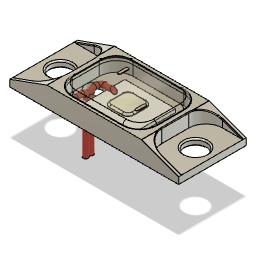
camera-imx335 (1) (Autodesk Fusion 360 archive; units mm, degrees)
design "LED light v3"
Autodesk Fusion 360 part; units mm, degrees
sketch "Sketch1" plane through (0, 0, 0) normal (0, 1, 0) x (1, 0, 0)
  line L0 (7.5, 6) -> (-7.5, 6)
  line L1 (-7.5, 6) -> (-7.5, -6)
  line L2 (-7.5, -6) -> (7.5, -6)
  line L3 (7.5, -6) -> (7.5, 6)
  line L4 (7.5, 6) -> (-7.5, -6) construction
  line L5 (-7.5, 6) -> (7.5, -6) construction
  dimension "d1" = 12
  dimension "d2" = 15
  constraint perpendicular L0 L1
  constraint parallel L0 L2
  constraint parallel L1 L3
  constraint horizontal L0
  constraint coincident L4 origin
  constraint coincident L5 origin
  measures "d1" distance of L0.end L1.end
  measures "d2" distance of L2.start L2.end L1
extrude "Extrude1" add sketch "Sketch1" along normal blind 1 makes body 1
sketch "Sketch2" plane through (0, 1, 0) normal (0, 1, 0) x (-1, 0, 0)
  line L0 (-7.5, 6) -> (-7.5, -6)
  line L1 (-7.5, -6) -> (7.5, -6)
  line L2 (7.5, -6) -> (7.5, 6)
  line L3 (7.5, 6) -> (-7.5, 6)
  line L4 (-3.55, -3.55) -> (3.55, -3.55)
  line L5 (3.55, -3.55) -> (3.55, 3.55)
  line L6 (3.55, 3.55) -> (-3.55, 3.55)
  line L7 (-3.55, 3.55) -> (-3.55, -3.55)
  line L8 (-3.55, -3.55) -> (3.55, 3.55) construction
  line L9 (3.55, -3.55) -> (-3.55, 3.55) construction
  dimension "d5" = 7.1
  dimension "d6" = 7.1
  constraint perpendicular L4 L5
  constraint parallel L4 L6
  constraint parallel L5 L7
  constraint horizontal L4
  constraint coincident L8 origin
  constraint coincident L9 origin
  measures "d5" distance of L5.end L6.end
  measures "d6" distance of L4.end L5.end
extrude "Extrude2" add sketch "Sketch2" along normal blind 0.6 separate body contours L4 L5 L6 L7 makes body 2
fillet "Fillet1" radius 1.7 4 edges at (3.55, 1.3, 3.55) (-3.55, 1.3, 3.55) (3.55, 1.3, -3.55) (-3.55, 1.3, -3.55) on bodies 2
fillet "Fillet2" radius 0.5 8 edges at (3.55, 1.6, 0) (3.0521, 1.6, 3.0521) (0, 1.6, 3.55) (-3.0521, 1.6, 3.0521) (-3.55, 1.6, 0) (-3.0521, 1.6, -3.0521) (0, 1.6, -3.55) (3.0521, 1.6, -3.0521) on bodies 2
sketch "Sketch3" plane through (0, 0, 0) normal (0, -1, 0) x (1, 0, 0)
  line L0 (7.5, -6) -> (7.5, 6)
  line L1 (7.5, 6) -> (-7.5, 6)
  line L2 (-7.5, 6) -> (-7.5, -6)
  line L3 (-7.5, -6) -> (7.5, -6)
  line L4 (25, 10) -> (-25, 10)
  line L5 (-25, 10) -> (-25, -10)
  line L6 (-25, -10) -> (25, -10)
  line L7 (25, -10) -> (25, 10)
  line L8 (25, 10) -> (-25, -10) construction
  line L9 (-25, 10) -> (25, -10) construction
  dimension "d11" = 50
  dimension "d12" = 20
  constraint perpendicular L4 L5
  constraint parallel L4 L6
  constraint parallel L5 L7
  constraint horizontal L4
  constraint coincident L8 origin
  constraint coincident L9 origin
  measures "d11" distance of L5.end L6.end
  measures "d12" distance of L4.end L5.end
extrude "Extrude3" add sketch "Sketch3" along normal blind 2 separate body contours L0 L1 L2 L3 | L4 L5 L6 L7 makes body 3
sketch "Sketch4" plane through (0, 0, 0) normal (0, 1, 0) x (-1, 0, 0)
  line L0 (-25, 10) -> (-25, -10)
  line L1 (-25, -10) -> (25, -10)
  line L2 (25, -10) -> (25, 10)
  line L3 (25, 10) -> (-25, 10)
  line L4 (12.5, 9) -> (-12.5, 9)
  line L5 (-12.5, 9) -> (-12.5, -9)
  line L6 (-12.5, -9) -> (12.5, -9)
  line L7 (12.5, -9) -> (12.5, 9)
  line L8 (12.5, 9) -> (-12.5, -9) construction
  line L9 (-12.5, 9) -> (12.5, -9) construction
  line L10 (-12.5, -9) -> (-14, -9)
  line L11 (12.5, -9) -> (14, -9)
  line L12 (14, -9) -> (25, -9)
  line L13 (25, -9) -> (25, 9)
  line L14 (25, 9) -> (14, 9)
  line L15 (14, 9) -> (14, -9)
  line L16 (-14, -9) -> (-25, -9)
  line L17 (-25, -9) -> (-25, 9)
  line L18 (-25, 9) -> (-14, 9)
  line L19 (-14, 9) -> (-14, -9)
  dimension "d15" = 25
  dimension "d16" = 18
  dimension "d18" = 1.5
  dimension "d19" = 1.5
  constraint perpendicular L4 L5
  constraint parallel L4 L6
  constraint parallel L5 L7
  constraint horizontal L4
  constraint coincident L8 origin
  constraint coincident L9 origin
  constraint horizontal L10
  constraint horizontal L11
  constraint horizontal L12
  constraint vertical L13
  constraint horizontal L14
  constraint vertical L15
  constraint coincident L2 L13.end
  constraint horizontal L16
  constraint vertical L17
  constraint horizontal L18
  constraint vertical L19
  constraint coincident L0 L17.end
  measures "d15" distance of L5.end L6.end
  measures "d16" distance of L4.end L5.end
  measures "d18" distance of L5.end L10.end
  measures "d19" distance of L6.end L11.end
extrude "Extrude4" add sketch "Sketch4" along normal blind 4 contours L0 L2 L3 L4 L5 L7 L10 L11 L14 L15 L18 L19 | L0 L1 L2 L6 L10 L11 L12 L16 bodies 3 1
fillet "Fillet3" radius 5 8 edges at (-12.5, 2, -9) (12.5, 2, -9) (12.5, 2, 9) (-12.5, 2, 9) (14, 2, 9) (14, 2, -9) (-14, 2, -9) (-14, 2, 9) on bodies 3
chamfer "Chamfer1" distance 11 distance2 4 4 edges at (-25, 4, -9.5) (-25, 4, 9.5) (25, 4, 9.5) (25, 4, -9.5) measured on face at (13.5, 4, 1.3333) measured on face at (13.5, 4, 1.3333) measured on face at (13.5, 4, 1.3333) measured on face at (13.5, 4, 1.3333) on bodies 3
sketch "Sketch6" plane through (0, 0, 0) normal (0, 1, 0) x (-1, 0, 0)
  arc A0 (-19, -9) -> (-14, -4) centre (-19, -4) ccw
  line L0 (-14, -4) -> (-14, 4)
  arc A1 (-14, 4) -> (-19, 9) centre (-19, 4) ccw
  line L1 (-19, 9) -> (-25, 9)
  line L2 (-25, 9) -> (-25, -9)
  line L3 (-25, -9) -> (-19, -9)
  line L4 (-25, 0) -> (-20, 0)
  line L5 (25, 9) -> (25, -9)
  line L6 (25, 0) -> (20, 0)
  circle A2 centre (20, 0) radius 3.25
  circle A3 centre (-20, 0) radius 3.25
  dimension "d25" = 6.5
  dimension "d26" = 6.5
  constraint midpoint L2 L4.start
  constraint perpendicular L0 L4
  constraint midpoint L5 L6.start
  constraint perpendicular L5 L6
  constraint coincident L6.end A2.centre
  constraint coincident L4.end A3.centre
  measures "d25" diameter of A2
  measures "d26" diameter of A3
extrude "Extrude5" cut sketch "Sketch6" against normal up to surface (2 mm away) contours A2 | A3 bodies 3 1
fillet "Fillet5" radius 0.2 22 edges at (11.0355, 4, -7.5355) (12.5, 4, 0) (11.0355, 4, 7.5355) (0, 4, 9) (-11.0355, 4, 7.5355) (-12.5, 4, 0) (-11.0355, 4, -7.5355) (0, 4, -9) (15.4645, 3.4675, -7.5355) (22, 1.0909, -9) (14, 4, 0) (22, 1.0909, 9) (15.4645, 3.4675, 7.5355) (-15.4645, 3.4675, 7.5355) (-22, 1.0909, 9) (-14, 4, 0) (-22, 1.0909, -9) (-15.4645, 3.4675, -7.5355) (14, 4, -7) (-14, 4, -7) (-14, 4, 7) (14, 4, 7) on bodies 3
sketch "Sketch7" plane through (0, 0, 0) normal (0, 1, 0) x (-1, 0, 0)
  arc A0 (12.5, 4) -> (7.5, 9) centre (7.5, 4) ccw
  line L0 (7.5, 9) -> (-7.5, 9)
  arc A1 (-7.5, 9) -> (-12.5, 4) centre (-7.5, 4) ccw
  line L1 (-12.5, 4) -> (-12.5, -4)
  arc A2 (-12.5, -4) -> (-7.5, -9) centre (-7.5, -4) ccw
  line L2 (-7.5, -9) -> (7.5, -9)
  arc A3 (7.5, -9) -> (12.5, -4) centre (7.5, -4) ccw
  line L3 (12.5, -4) -> (12.5, 4)
  circle A4 centre (10, 0) radius 2.5
  constraint tangent L3 A4
extrude "Extrude6" cut sketch "Sketch7" against normal up to surface (2 mm away) contours A4 bodies 3 1
fillet "Fillet4" radius 0.4 5 edges at (-16.9699, 0, 1.1753) (-16.9699, -2, -1.1753) (-7.6692, -2, -0.904) (23.0301, -2, -1.1753) (23.0301, 0, 1.1753) on bodies 3
sketch "Sketch8" plane through (0, 1, 0) normal (0, 1, 0) x (-1, 0, 0)
  line L0 (-7.5, 6) -> (-7.5, -6)
  line L1 (-7.5, -6) -> (7.5, -6)
  line L2 (7.5, -6) -> (7.5, 6)
  line L3 (7.5, 6) -> (-7.5, 6)
  line L4 (0, 0) -> (6, 0) construction
  line L5 (6, 0) -> (6, -3.4) construction
  line L6 (5.5, -2.3) -> (5.5, -4.5)
  arc A0 (5.5, -4.5) -> (6.5, -4.5) centre (6, -4.5) ccw
  line L7 (6.5, -4.5) -> (6.5, -2.3)
  arc A1 (6.5, -2.3) -> (5.5, -2.3) centre (6, -2.3) ccw
  line L8 (6, -2.3) -> (6, -4.5) construction
  point P0 (6, -3.4)
  dimension "d34" = 6
  dimension "d35" = 90
  dimension "d36" = 3.4
  constraint coincident L4.start origin
  constraint horizontal L4
  constraint tangent L6 A0
  constraint tangent A0 L7
  constraint parallel L6 L7
  constraint tangent L7 A1
  constraint tangent L6 A1
  constraint parallel L5 L8
  constraint midpoint L8 P0
  measures "d34" distance of L4.start L4.end
  measures "d35" angle of L4 L5
  measures "d36" distance of L4.end P0
extrude "Extrude7" add sketch "Sketch8" along normal blind 0.1 separate body contours L6 A0 L7 A1 makes body 4
fillet "Fillet6" radius 0.1 4 edges at (-6.5, 1.1, -3.4) (-6, 1.1, -1.8) (-5.5, 1.1, -3.4) (-6, 1.1, -5) on bodies 4
pattern_circular "C-Pattern1" count 2 over 360 about axis through (0, 1.75, 0) along (0, 1, 0) of "Extrude7", "Fillet6" makes body 5
sketch "Sketch9" plane through (0, 0, 0) normal (0, 1, 0) x (-1, 0, 0)
  arc A0 (12.5, 4) -> (7.5, 9) centre (7.5, 4) ccw
  line L0 (7.5, 9) -> (-7.5, 9)
  arc A1 (-7.5, 9) -> (-12.5, 4) centre (-7.5, 4) ccw
  line L1 (-12.5, 4) -> (-12.5, -4)
  arc A2 (-12.5, -4) -> (-7.5, -9) centre (-7.5, -4) ccw
  line L2 (-7.5, -9) -> (7.5, -9)
  arc A3 (7.5, -9) -> (12.5, -4) centre (7.5, -4) ccw
  line L3 (12.5, -4) -> (12.5, 0)
  circle A4 centre (10, 0) radius 2.5
  line L4 (12.5, 0) -> (12.5, 4)
  circle A5 centre (10, -0.75) radius 0.75
  circle A6 centre (10, 0.75) radius 0.75
  dimension "d42" = 1.5
  dimension "d43" = 1.5
  constraint coincident A4.centre A5
  constraint coincident A4.centre A6
  measures "d42" diameter of A5
  measures "d43" diameter of A6
extrude "Extrude8" add sketch "Sketch9" against normal blind 15 separate body contours A6 makes body 6
extrude "Extrude9" add sketch "Sketch9" against normal blind 15 separate body contours A5 makes body 7
extrude "Extrude10" add sketch "Sketch9" along normal blind 0.8 contours A5 bodies 7 6
sketch "Sketch11" plane through (0, 0.8, 0) normal (0, 1, 0) x (-1, 0, 0)
  line L0 (9, 1.7) -> (11, 1.7) construction
  line L1 (9, -1.7) -> (11, -1.7) construction
  circle A0 centre (10, -0.75) radius 0.75
  constraint horizontal L0
  constraint horizontal L1
revolve "Revolve3" add 1 faces at (-9.6465, 0.8, -0.5183) angle 90 about axis through (-9, 0.8, -1.7) along (-1, 0, 0) on bodies 7 bodies 7
extrude "Extrude12" add 1 faces at (-9.4778, 1.7363, -1.7) along direction (0, 0, -1) blind 1 on bodies 7 bodies 7
extrude "Extrude14" add 1 faces at (-10.0834, 0, 0.9807) along direction (0, 1, 0) blind 0.8 on bodies 7 bodies 7
sketch "Sketch12" plane through (0, 0, -2.7) normal (0, 0, -1) x (-1, 0, 0)
  circle A0 centre (10, 1.75) radius 0.75
  line L0 (9, 1.5) -> (9, 3)
  constraint vertical L0
revolve "Revolve5" add sketch "Sketch12" angle 90 about axis through (-9, 1.5, -2.7) along (0, -1, 0) bodies 7
extrude "Extrude13" add 1 faces at (-9, 2.2722, -3.6024) along direction (1, 0, 0) blind 3.4 on bodies 7 bodies 7
sketch "Sketch15" plane through (0, 0, 0) normal (0, 0, 1) x (1, 0, 0)
  line L0 (-5.6, 1.2) -> (-7.3678, 2.9678)
  line L1 (-5.6, 1.2) -> (-3.1, 1.2) construction
  line L2 (-7.3678, 2.9678) -> (-5.5, 2.9678)
  line L3 (-5.5, 2.9678) -> (-5.5, 1.2)
  line L4 (-5.5, 1.2) -> (-5.6, 1.2)
  dimension "d63" = 135
  dimension "d64" = 2.5
  constraint horizontal L1
  constraint horizontal L2
  constraint coincident L1 L3.end
  constraint perpendicular L1 L3
  measures "d63" angle of L0 L1
  measures "d64" distance of L0.start L0.end
extrude "Extrude15" cut sketch "Sketch15" against normal blind 5 bodies 7
revolve "Revolve6" add 1 faces at (-10.0834, 0.8, 0.9807) angle 90 about axis through (-9, 0.8, 1.7) along (1, 0, 0) on bodies 7 bodies 7
extrude "Extrude16" add 1 faces at (-9.588, 1.4691, 1.7) along direction (0, 0, 1) blind 2 on bodies 7 bodies 7
sketch "Sketch16" plane through (0, 0, 3.7) normal (0, 0, 1) x (1, 0, 0)
  circle A0 centre (-10, 1.75) radius 0.75
  line L0 (-9, 1) -> (-9, 2.5)
  line L1 (-9, 1) -> (-9, 2.7)
  constraint coincident L0 L1.end
  constraint parallel L0 L1
revolve "Revolve7" add sketch "Sketch16" angle 90 about axis through (-9, 1, 3.7) along (0, 1, 0) bodies 7
extrude "Extrude17" add 1 faces at (-9, 1.3727, 4.4528) along direction (1, 0, 0) blind 15.5 on bodies 7 bodies 7
sketch "Sketch17" plane through (0, 0, 0) normal (0, 0, 1) x (1, 0, 0)
  line L0 (6.5, 1.1829) -> (4.7322, 2.9506)
  line L1 (6.5, 1.1829) -> (9, 1.1829) construction
  line L2 (4.7322, 2.9506) -> (7, 2.9506)
  line L3 (7, 2.9506) -> (7, 1.1829)
  line L4 (7, 1.1829) -> (6.5, 1.1829)
  dimension "d73" = 135
  dimension "d74" = 2.5
  constraint horizontal L1
  constraint horizontal L2
  constraint coincident L1 L3.end
  constraint perpendicular L1 L3
  measures "d73" angle of L0 L1
  measures "d74" distance of L0.start L0.end
extrude "Extrude18" cut sketch "Sketch17" along normal blind 6 bodies 7
sketch "Sketch18" plane through (0, 0, 0) normal (0, 1, 0) x (-1, 0, 0)
  arc A0 (12.5, 4) -> (7.5, 9) centre (7.5, 4) ccw
  line L0 (7.5, 9) -> (-7.5, 9)
  arc A1 (-7.5, 9) -> (-12.5, 4) centre (-7.5, 4) ccw
  line L1 (-12.5, 4) -> (-12.5, -4)
  arc A2 (-12.5, -4) -> (-7.5, -9) centre (-7.5, -4) ccw
  line L2 (-7.5, -9) -> (7.5, -9)
  arc A3 (7.5, -9) -> (12.5, -4) centre (7.5, -4) ccw
  line L3 (12.5, -4) -> (12.5, 0)
  circle A4 centre (10, 0) radius 2.5
  line L4 (12.5, 0) -> (12.5, 4)
extrude "Extrude19" add sketch "Sketch18" along normal blind 2 from surface at 3 separate body contours A4 | A0 L0 A1 L1 A2 L2 A3 L3 L4 makes body 8
fillet "Fillet7" radius 1 8 edges at (12.5, 5, 0) (11.0355, 5, -7.5355) (0, 5, -9) (-11.0355, 5, -7.5355) (-12.5, 5, 0) (-11.0355, 5, 7.5355) (0, 5, 9) (11.0355, 5, 7.5355) on bodies 8
move_body "Move1" bodies 3 to x (1, 0, 0) y (0, 1, 0) z (0, 0, 1) at (33.2468, 0, 148.1523)
move_body "Move2" bodies 8 to x (1, 0, 0) y (0, 1, 0) z (0, 0, 1) at (33.2468, 0, 148.1523)
move_body "Move3" bodies 2 to x (1, 0, 0) y (0, 1, 0) z (0, 0, 1) at (33.2468, 0, 148.1523)
move_body "Move4" bodies 1 to x (1, 0, 0) y (0, 1, 0) z (0, 0, 1) at (33.83, 0, 148.1523)
move_body "Move5" bodies 7 to x (1, 0, 0) y (0, 1, 0) z (0, 0, 1) at (34.4133, 0, 151.0686)
move_body "Move6" bodies 3 2 8 1 7 to x (1, 0, 0) y (0, 1, 0) z (0, 0, 1) at (0, -63.5772, 0.5833)
move_body "Move7" bodies 5 4 to x (1, 0, 0) y (0, 1, 0) z (0, 0, 1) at (32.8312, -60.6608, 147.1306)
move_body "Move8" bodies 5 2 8 4 1 3 7 to x (1, 0, 0) y (0, 1, 0) z (0, 0, 1) at (-0.5833, -6.416, 0)
equation "d34 = ( 12 / 2 ) * 1 mm"
equation "d36 = ( 6.8 / 2 ) * 1 mm"
